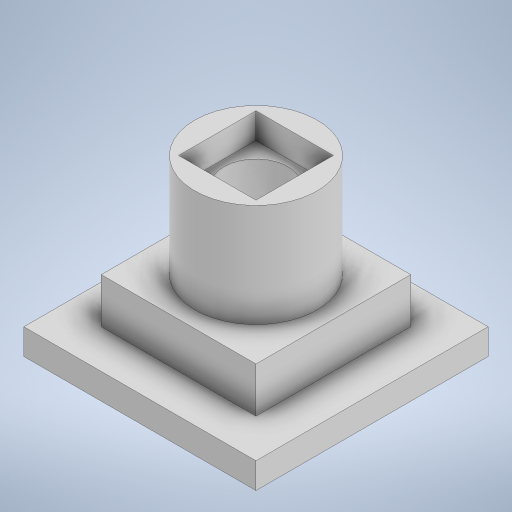
# Autodesk Inventor part: HexPivot
Saved by Autodesk Inventor 2024 (Build 280153000, 153)
## iProperties
Created: 2026-02-04
Part Number: HexPivot
Material: Generic
Document SubType Name: Modeling
Designer: Liam
Density: 1 g/cm^3
Appearance: Default
Author: Liam
Autodesk Inventor part; units mm, degrees
ref_plane "YZ Plane" through (0, 0, 0) normal (1, 0, 0) x (0, 1, 0)
ref_plane "XZ Plane" through (0, 0, 0) normal (0, 1, 0) x (-1, 0, 0)
ref_plane "XY Plane" through (0, 0, 0) normal (0, 0, 1) x (1, 0, 0)
sketch "Sketch1" plane through (0, 0, 0) normal (0, 1, 0) x (-1, 0, 0)
  circle A0 centre (0, 0) radius 2.5
  circle A1 centre (0, 0) radius 4.75
  line L0 (3, 3) -> (-3, 3)
  line L1 (-3, 3) -> (-3, -3)
  line L2 (-3, -3) -> (3, -3)
  line L3 (3, -3) -> (3, 3)
  line L4 (3, 3) -> (-3, -3) construction
  line L5 (-3, 3) -> (3, -3) construction
  line L6 (6, 6) -> (-6, 6)
  line L7 (-6, 6) -> (-6, -6)
  line L8 (-6, -6) -> (6, -6)
  line L9 (6, -6) -> (6, 6)
  line L10 (6, 6) -> (-6, -6) construction
  line L11 (-6, 6) -> (6, -6) construction
  line L12 (9, 9) -> (-9, 9)
  line L13 (-9, 9) -> (-9, -9)
  line L14 (-9, -9) -> (9, -9)
  line L15 (9, -9) -> (9, 9)
  line L16 (9, 9) -> (-9, -9) construction
  line L17 (-9, 9) -> (9, -9) construction
  dimension "d9" = 5
  dimension "d10" = 9.5
  dimension "d11" = 6
  dimension "d12" = 6
  dimension "d13" = 12
  dimension "d14" = 12
  dimension "d15" = 18
  constraints: 36 end point, 6 midpoint, 6 parallel, 3 horizontal, 3 perpendicular, 2 centre point, 2 coincident, 1 point on line
  measures "d9" diameter of A0
  measures "d10" diameter of A1
  measures "d11" distance of L1.end L2.end
  measures "d12" distance of L2.end L0.start
  measures "d13" distance of L8.end L6.start
  measures "d14" distance of L7.end L8.end
  measures "d15" distance of L13.end L14.end
extrude "Extrusion1" add sketch "Sketch1" against normal blind 2 contours A0 | A1 | L3 L2 L1 L0 | L9 L8 L7 L6 | L15 L14 L13 L12
extrude "Extrusion2" add sketch "Sketch1" along normal blind 3.5 contours L9 L8 L7 L6
extrude "Extrusion3" add sketch "Sketch1" along normal blind 11.5 contours A1
extrude "Extrusion4" add sketch "Sketch1" along normal blind 9.5 contours L3 L2 L1 L0
extrude "Extrusion5" add sketch "Sketch1" along normal blind 4.5 contours A0
equation "\"d13\" = PIVOT_SQUARE"
equation "\"d14\" = PIVOT_SQUARE"
equation "\"PIVOT_SQUARE\" = 12"
body "Solid1"
